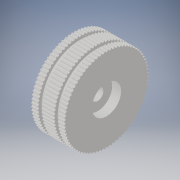
# Autodesk Inventor part: correct_wheel
Saved by Autodesk Inventor 2019 (Build 230136000, 136)
## iProperties
Created: 2017-11-06
Part Number: correct_wheel
Material: Generic
Document SubType Name: Modeling
Designer: kcmat
Density: 1 g/cm^3
Appearance: Default
Author: kcmat
Autodesk Inventor part; units mm, degrees
ref_plane "YZ Plane" through (0, 0, 0) normal (1, 0, 0) x (0, 1, 0)
ref_plane "XZ Plane" through (0, 0, 0) normal (0, 1, 0) x (-1, 0, 0)
ref_plane "XY Plane" through (0, 0, 0) normal (0, 0, 1) x (1, 0, 0)
sketch "Sketch1" plane through (0, 0, 0) normal (1, 0, 0) x (0, 1, 0)
  circle A0 centre (0, 0) radius 25.4
  circle A1 centre (0, 0) radius 4.445
  dimension "d3" = 8.89
  constraints: 2 centre point, 1 coincident
  measures "d3" diameter of A1
extrude "Extrusion1" add sketch "Sketch1" along normal blind 25.4
sketch "Sketch2" plane through (0, 0, 0) normal (-1, 0, 0) x (0, 0, 1)
  circle A0 centre (0, 0) radius 10.9855
  dimension "d6" = 21.971
  constraints: 1 centre point, 1 coincident
  measures "d6" diameter of A0
extrude "Extrusion2" cut sketch "Sketch2" against normal blind 6.858
sketch "Sketch3" plane through (25.4, 0, 0) normal (1, 0, 0) x (0, 0, -1)
  circle A0 centre (0, 0) radius 10.9855
  dimension "d9" = 21.971
  constraints: 1 centre point, 1 coincident
  measures "d9" diameter of A0
extrude "Extrusion3" cut sketch "Sketch3" against normal blind 6.858
sketch "Sketch5" plane through (25.4, 0, 0) normal (1, 0, 0) x (0, 0, -1)
  circle A0 centre (0, 0) radius 4.445 projected
  circle A1 centre (0, 0) radius 11.176
  dimension "d48" = 22.352
  constraints: 1 centre point, 1 coincident
  measures "d48" diameter of A1
extrude "Extrusion8" cut sketch "Sketch5" against normal up to surface (6.858 mm away)
sketch "Sketch8" plane through (25.4, 0, 0) normal (1, 0, 0) x (0, 0, -1)
  circle A0 centre (0, 0) radius 32.5
  circle A1 centre (0, 0) radius 11.176 projected
  circle A2 centre (0, 0) radius 25.4 projected
  dimension "d54" = 65
  constraints: 1 centre point, 1 coincident
  measures "d54" diameter of A0
extrude "Extrusion10" add sketch "Sketch8" against normal blind 25.4 contours A0
sketch "Sketch9" plane through (25.4, 0, 0) normal (1, 0, 0) x (0, 0, -1)
  circle A0 centre (0, 0) radius 32.5 projected
  circle A1 centre (0, 32.5) radius 1
  circle A2 centre (-2.5499, 32.3998) radius 1
  circle A3 centre (-5.0841, 32.0999) radius 1
  circle A4 centre (-7.587, 31.602) radius 1
  circle A5 centre (-10.0431, 30.9093) radius 1
  circle A6 centre (-12.4372, 30.0261) radius 1
  circle A7 centre (-14.7547, 28.9577) radius 1
  circle A8 centre (-16.9812, 27.7108) radius 1
  circle A9 centre (-19.103, 26.2931) radius 1
  circle A10 centre (-21.1071, 24.7132) radius 1
  circle A11 centre (-22.981, 22.981) radius 1
  circle A12 centre (-24.7132, 21.1071) radius 1
  circle A13 centre (-26.2931, 19.103) radius 1
  circle A14 centre (-27.7108, 16.9812) radius 1
  circle A15 centre (-28.9577, 14.7547) radius 1
  circle A16 centre (-30.0261, 12.4372) radius 1
  circle A17 centre (-30.9093, 10.0431) radius 1
  circle A18 centre (-31.602, 7.587) radius 1
  circle A19 centre (-32.0999, 5.0841) radius 1
  circle A20 centre (-32.3998, 2.5499) radius 1
  circle A21 centre (-32.5, 0) radius 1
  circle A22 centre (-32.3998, -2.5499) radius 1
  circle A23 centre (-32.0999, -5.0841) radius 1
  circle A24 centre (-31.602, -7.587) radius 1
  circle A25 centre (-30.9093, -10.0431) radius 1
  circle A26 centre (-30.0261, -12.4372) radius 1
  circle A27 centre (-28.9577, -14.7547) radius 1
  circle A28 centre (-27.7108, -16.9812) radius 1
  circle A29 centre (-26.2931, -19.103) radius 1
  circle A30 centre (-24.7132, -21.1071) radius 1
  circle A31 centre (-22.981, -22.981) radius 1
  circle A32 centre (-21.1071, -24.7132) radius 1
  circle A33 centre (-19.103, -26.2931) radius 1
  circle A34 centre (-16.9812, -27.7108) radius 1
  circle A35 centre (-14.7547, -28.9577) radius 1
  circle A36 centre (-12.4372, -30.0261) radius 1
  circle A37 centre (-10.0431, -30.9093) radius 1
  circle A38 centre (-7.587, -31.602) radius 1
  circle A39 centre (-5.0841, -32.0999) radius 1
  circle A40 centre (-2.5499, -32.3998) radius 1
  circle A41 centre (0, -32.5) radius 1
  circle A42 centre (2.5499, -32.3998) radius 1
  circle A43 centre (5.0841, -32.0999) radius 1
  circle A44 centre (7.587, -31.602) radius 1
  circle A45 centre (10.0431, -30.9093) radius 1
  circle A46 centre (12.4372, -30.0261) radius 1
  circle A47 centre (14.7547, -28.9577) radius 1
  circle A48 centre (16.9812, -27.7108) radius 1
  circle A49 centre (19.103, -26.2931) radius 1
  circle A50 centre (21.1071, -24.7132) radius 1
  circle A51 centre (22.981, -22.981) radius 1
  circle A52 centre (24.7132, -21.1071) radius 1
  circle A53 centre (26.2931, -19.103) radius 1
  circle A54 centre (27.7108, -16.9812) radius 1
  circle A55 centre (28.9577, -14.7547) radius 1
  circle A56 centre (30.0261, -12.4372) radius 1
  circle A57 centre (30.9093, -10.0431) radius 1
  circle A58 centre (31.602, -7.587) radius 1
  circle A59 centre (32.0999, -5.0841) radius 1
  circle A60 centre (32.3998, -2.5499) radius 1
  circle A61 centre (32.5, 0) radius 1
  circle A62 centre (32.3998, 2.5499) radius 1
  circle A63 centre (32.0999, 5.0841) radius 1
  circle A64 centre (31.602, 7.587) radius 1
  circle A65 centre (30.9093, 10.0431) radius 1
  circle A66 centre (30.0261, 12.4372) radius 1
  circle A67 centre (28.9577, 14.7547) radius 1
  circle A68 centre (27.7108, 16.9812) radius 1
  circle A69 centre (26.2931, 19.103) radius 1
  circle A70 centre (24.7132, 21.1071) radius 1
  circle A71 centre (22.981, 22.981) radius 1
  circle A72 centre (21.1071, 24.7132) radius 1
  circle A73 centre (19.103, 26.2931) radius 1
  circle A74 centre (16.9812, 27.7108) radius 1
  circle A75 centre (14.7547, 28.9577) radius 1
  circle A76 centre (12.4372, 30.0261) radius 1
  circle A77 centre (10.0431, 30.9093) radius 1
  circle A78 centre (7.587, 31.602) radius 1
  circle A79 centre (5.0841, 32.0999) radius 1
  circle A80 centre (2.5499, 32.3998) radius 1
  dimension "d57" = 2
  dimension "d60" = 360
  constraints: 80 centre point, 1 vertical alignment, 162 other
  measures "d57" diameter of A1
extrude "Extrusion11" cut sketch "Sketch9" against normal up to surface (25.4 mm away) contours A0 A61 | A0 A61 | A62 A0 | A0 A62 | A60 A0 | A0 A60 | A63 A0 | A0 A63 | A59 A0 | A0 A59 | A64 A0 | A0 A64 | A58 A0 | A0 A58 | A65 A0 | A0 A65 | A57 A0 | A0 A57 | A66 A0 | A0 A66 | A56 A0 | A0 A56 | A67 A0 | A0 A67 | A55 A0 | A0 A55 | A68 A0 | A0 A68 | A54 A0 | A0 A54 | A69 A0 | A0 A69 | A53 A0 | A0 A53 | A70 A0 | A0 A70 | A52 A0 | A0 A52 | A71 A0 | A0 A71 | A51 A0 | A0 A51 | A72 A0 | A0 A72 | A50 A0 | A0 A50 | A73 A0 | A0 A73 | A49 A0 | A0 A49 | A74 A0 | A0 A74 | A48 A0 | A0 A48 | A75 A0 | A0 A75 | A47 A0 | A0 A47 | A76 A0 | A0 A76 | A46 A0 | A0 A46 | A77 A0 | A0 A77 | A45 A0 | A0 A45 | A78 A0 | A0 A78 | A44 A0 | A0 A44 | A79 A0 | A0 A79 | A43 A0 | A0 A43 | A80 A0 | A0 A80 | A42 A0 | A0 A42 | A1 A0 | A0 A1 | A41 A0 | A0 A41 | A2 A0 | A0 A2 | A40 A0 | A0 A40 | A3 A0 | A0 A3 | A39 A0 | A0 A39 | A4 A0 | A0 A4 | A38 A0 | A0 A38 | A5 A0 | A0 A5 | A37 A0 | A0 A37 | A6 A0 | A0 A6 | A36 A0 | A0 A36 | A7 A0 | A0 A7 | A35 A0 | A0 A35 | A8 A0 | A0 A8 | A34 A0 | A0 A34 | A9 A0 | A0 A9 | A33 A0 | A0 A33 | A10 A0 | A0 A10 | A32 A0 | A0 A32 | A11 A0 | A0 A11 | A31 A0 | A0 A31 | A12 A0 | A0 A12 | A30 A0 | A0 A30 | A13 A0 | A0 A13 | A29 A0 | A0 A29 | A14 A0 | A0 A14 | A28 A0 | A0 A28 | A15 A0 | A0 A15 | A27 A0 | A0 A27 | A16 A0 | A0 A16 | A26 A0 | A0 A26 | A17 A0 | A0 A17 | A25 A0 | A0 A25 | A18 A0 | A0 A18 | A24 A0 | A0 A24 | A19 A0 | A0 A19 | A23 A0 | A0 A23 | A20 A0 | A0 A20 | A22 A0 | A0 A22 | A21 A0 | A0 A21
sketch "Sketch10" plane through (0, 0, 0) normal (0, 0, 1) x (1, 0, 0)
  line L0 (0, 32.4846) -> (25.4, 32.4846) projected
  line L1 (5, 32.4846) -> (8, 32.4846)
  line L2 (8, 32.4846) -> (8, 29.4846)
  line L3 (8, 29.4846) -> (5, 29.4846)
  line L4 (5, 29.4846) -> (5, 32.4846)
  line L5 (20.4, 32.4846) -> (17.4, 32.4846)
  line L6 (17.4, 32.4846) -> (17.4, 29.4846)
  line L7 (17.4, 29.4846) -> (20.4, 29.4846)
  line L8 (20.4, 29.4846) -> (20.4, 32.4846)
  line L9 (0, 31.5) -> (0, 32.4846) projected
  line L10 (25.4, 32.4846) -> (25.4, 31.5) projected
  line L11 (0, 0) -> (31.1419, 0) construction
  line L12 (5, 32.4846) -> (8, 32.4846)
  line L13 (8, 32.4846) -> (8, 33.0264)
  line L14 (8, 33.0264) -> (5, 33.0264)
  line L15 (5, 33.0264) -> (5, 32.4846)
  line L16 (17.4, 32.4846) -> (20.4, 32.4846)
  line L17 (20.4, 32.4846) -> (20.4, 33.0264)
  line L18 (20.4, 33.0264) -> (17.4, 33.0264)
  line L19 (17.4, 33.0264) -> (17.4, 32.4846)
  dimension "d64" = 3
  dimension "d65" = 3
  dimension "d66" = 5
  dimension "d67" = 5
  dimension "d68" = 3
  constraints: 34 end point, 8 parallel, 5 horizontal, 4 perpendicular, 4 point on line
  measures "d64" distance of L1.end L2.end
  measures "d65" distance of L2.end L3.end
  measures "d66" distance between parallel lines of L4 L9
  measures "d67" distance between parallel lines of L10 L8
  measures "d68" distance of L6.end L7.end
revolve "Revolution2" cut sketch "Sketch10" angle 360 about axis through (0, 0, 0) along (1, 0, 0)
body "Solid1"
